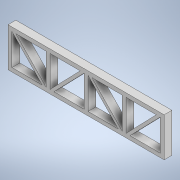
# Autodesk Inventor part: Kratownica
Saved by Autodesk Inventor 2021 (Build 250183000, 183)
## iProperties
Created: 2020-04-11
Part Number: Kratownica
Material: Ogólny
Document SubType Name: Modeling
Designer: dyrag
Density: 1 g/cm^3
Appearance: Domyślna
Author: dyrag
Autodesk Inventor part; units mm, degrees
ref_plane "YZ Plane" through (0, 0, 0) normal (1, 0, 0) x (0, 1, 0)
ref_plane "XZ Plane" through (0, 0, 0) normal (0, 1, 0) x (-1, 0, 0)
ref_plane "XY Plane" through (0, 0, 0) normal (0, 0, 1) x (1, 0, 0)
sketch "Szkic1" plane through (0, 0, 0) normal (0, 0, 1) x (1, 0, 0)
  line L0 (0, 0) -> (200, 0)
  line L1 (0, 0) -> (200, 0)
  line L2 (200, 0) -> (200, 50)
  line L3 (200, 50) -> (0, 50)
  line L4 (0, 50) -> (0, 0)
  line L5 (0, 0) -> (10, 0)
  line L6 (200, 50) -> (195, 50)
  line L7 (200, 50) -> (200, 45)
  line L8 (200, 50) -> (195, 50)
  line L9 (200, 50) -> (200, 45)
  line L10 (195, 45) -> (195, 5)
  line L11 (195, 5) -> (156.25, 5)
  line L12 (5, 5) -> (5, 45)
  line L13 (102.5, 45) -> (102.5, 5)
  line L14 (97.5, 45) -> (97.5, 5)
  line L15 (53.75, 45) -> (53.75, 5)
  line L16 (48.75, 45) -> (48.75, 5)
  line L17 (151.25, 45) -> (151.25, 5)
  line L18 (146.25, 45) -> (146.25, 5)
  line L19 (10, 45) -> (48.75, 5)
  line L20 (43.75, 5) -> (5, 45)
  line L21 (58.75, 5) -> (97.5, 45)
  line L22 (92.5, 45) -> (53.75, 5)
  line L23 (107.5, 45) -> (146.25, 5)
  line L24 (141.25, 5) -> (102.5, 45)
  line L25 (156.25, 5) -> (195, 45)
  line L26 (151.25, 5) -> (190, 45)
  line L27 (10, 45) -> (48.75, 45)
  line L28 (53.75, 45) -> (92.5, 45)
  line L29 (107.5, 45) -> (146.25, 45)
  line L30 (151.25, 45) -> (190, 45)
  line L31 (43.75, 5) -> (5, 5)
  line L32 (97.5, 5) -> (58.75, 5)
  line L33 (141.25, 5) -> (102.5, 5)
  dimension "d2" = 50
  constraints: 68 end point, 32 perpendicular, 10 point on line, 5 parallel, 4 collinear, 3 horizontal
  measures "d2" distance of L0.end L2.end
extrude "Wyciągnięcie proste1" add sketch "Szkic1" along normal blind 10
